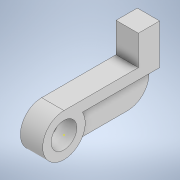
# Autodesk Inventor part: ServoHorn
Saved by Autodesk Inventor 2020 (Build 240168000, 168)
## iProperties
Created: 2020-06-08
Part Number: ServoHorn
Material: Generic
Document SubType Name: Modeling
Designer: Brandon
Density: 1 g/cm^3
Appearance: Default
Author: Brandon
Autodesk Inventor part; units mm, degrees
ref_plane "YZ Plane" through (0, 0, 0) normal (1, 0, 0) x (0, 1, 0)
ref_plane "XZ Plane" through (0, 0, 0) normal (0, 1, 0) x (-1, 0, 0)
ref_plane "XY Plane" through (0, 0, 0) normal (0, 0, 1) x (1, 0, 0)
sketch "Sketch1" plane through (0, 0, 0) normal (1, 0, 0) x (0, 1, 0)
  circle A0 centre (0, 0) radius 3.0734
  line L0 (5.08, 5.08) -> (-5.08, 5.08)
  line L1 (-5.08, 5.08) -> (-5.08, -22.86)
  line L2 (-5.08, -22.86) -> (5.08, -22.86)
  line L3 (5.08, -22.86) -> (5.08, 5.08)
  line L4 (-5.08, -22.86) -> (12.192, -22.86)
  line L5 (12.192, -22.86) -> (12.192, -17.78)
  line L6 (12.192, -17.78) -> (-5.08, -17.78)
  line L7 (-5.08, -17.78) -> (-5.08, -22.86)
  point P0 (5.08, -17.78)
  point P1 (5.08, -22.86)
  dimension "d0" = 6.1468
  dimension "d1" = 5.08
  dimension "d2" = 5.08
  dimension "d3" = 5.08
  dimension "d4" = 22.86
  dimension "d5" = 5.08
  dimension "d6" = 7.112
  constraints: 16 end point, 4 parallel, 2 horizontal, 2 perpendicular, 1 centre point, 1 coincident
  measures "d0" diameter of A0
  measures "d1" distance from line of point (0, 0) L3
  measures "d2" distance from line of point (0, 0) L1
  measures "d3" distance from line of point (0, 0) L0
  measures "d4" distance from line of point (0, 0) L2
  measures "d5" distance of L4.end L5.end
  measures "d6" distance between parallel lines of L3 L5
extrude "Extrusion1" add sketch "Sketch1" along normal blind 5.334
sketch "Sketch2" plane through (0, 0, 0) normal (-1, 0, 0) x (0, 0, 1)
  circle A0 centre (0, 0) radius 1.5875
  circle A1 centre (0, 0) radius 3.4736
  dimension "d9" = 3.175
  constraints: 2 centre point, 2 coincident
  measures "d9" diameter of A0
extrude "Extrusion2" add sketch "Sketch2" against normal blind 5.334
fillet "Fillet1" radius 5.08 3 edges at (2.667, -5.08, -22.86) (2.667, 5.08, 5.08) (2.667, -5.08, 5.08)
sketch "Sketch3" plane through (5.334, 0, 0) normal (1, 0, 0) x (0, 0, -1)
  point P0 (0, 0)
sketch "Sketch4" plane through (5.334, 0, 0) normal (1, 0, 0) x (0, 0, -1)
  circle A0 centre (0, 0) radius 5.08
  line L0 (5.08, 0) -> (23.4096, 0)
  line L1 (23.4096, 0) -> (23.4096, -6.5655)
  line L2 (23.4096, -6.5655) -> (5.08, -6.5655)
  line L3 (5.08, -6.5655) -> (5.08, 0)
  line L4 (0, -5.08) -> (17.78, -5.08) projected
  line L5 (0, -5.08) -> (4.9426, -5.08)
  point P0 (5.08, -5.08)
  constraints: 10 end point, 2 parallel, 1 centre point, 1 coincident, 1 horizontal, 1 perpendicular, 1 point on circle, 1 point on line
extrude "Extrusion3" cut sketch "Sketch4" against normal blind 2.54 contours L3 L4 A0 | L0 L1 L2 L3
chamfer "Chamfer1" distance 2.54 angle 45 1 edges at (5.334, 0, -13.97)
sketch "Sketch6" plane through (5.334, 0, 0) normal (1, 0, 0) x (0, 0, -1)
  circle A0 centre (0, 0) radius 3.0734
  dimension "d30" = 6.1468
  constraints: 1 centre point, 1 coincident
  measures "d30" diameter of A0
extrude "Extrusion5" cut sketch "Sketch6" against normal blind 4.064 draft -4
body "Solid1"
